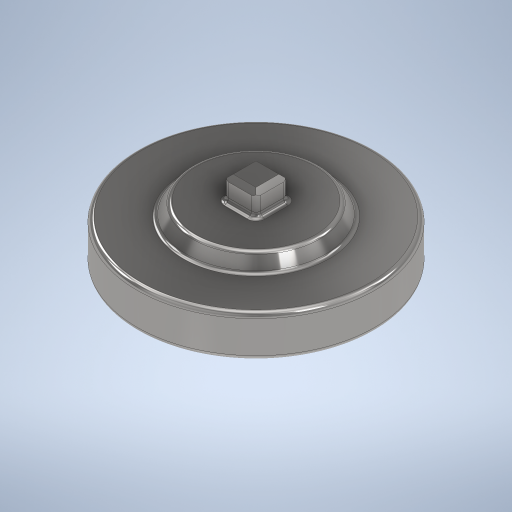
# Autodesk Inventor part: Disc
Saved by Autodesk Inventor 2024 (Build 280153000, 153)
## iProperties
Created: 2024-03-23
Part Number: Disc
Material: Generic
Document SubType Name: Sheet Metal
Designer: MSI-C
Density: 1 g/cm^3
Sheet Metal Rule: Default_mm
Appearance: Steel - Polished
Mass: 22.3559 g
Surface Area: 62.1848 cm^2
Volume: 22.3559 cm^3
Author: MSI-C
Autodesk Inventor part; units mm, degrees
ref_plane "YZ Plane" through (0, 0, 0) normal (1, 0, 0) x (0, 1, 0)
ref_plane "XZ Plane" through (0, 0, 0) normal (0, 1, 0) x (-1, 0, 0)
ref_plane "XY Plane" through (0, 0, 0) normal (0, 0, 1) x (1, 0, 0)
sketch "Sketch1" plane through (0, 0, 0) normal (0, 0, 1) x (1, 0, 0)
  line L0 (0, 0) -> (-5, 0)
  line L1 (-5, 0) -> (-5, 14)
  line L2 (-5, 14) -> (-26, 14)
  line L3 (-26, 14) -> (-26, 23)
  line L4 (-26, 23) -> (-15.5, 23)
  line L5 (-15.5, 23) -> (-13.5, 26)
  line L6 (-13.5, 26) -> (0, 26)
  line L7 (0, 26) -> (0, 0) construction
  line L8 (0, 26) -> (0, 0)
  dimension "d0" = 5
  dimension "d1" = 14
  dimension "d2" = 9
  dimension "d4" = 3
  dimension "d5" = 13.5
  dimension "d6" = 15.5
  dimension "d7" = 26
  dimension "d8" = 26
  constraints: 18 end point, 5 perpendicular, 2 horizontal, 2 vertical, 1 point on line
  measures "d0" distance of L0.start L0.end
  measures "d1" distance of L0.end L1.end
  measures "d2" distance of L2.end L3.end
  measures "d4" vertical distance of L4.end L5.end
  measures "d5" distance of L5.end L6.end
  measures "d6" horizontal distance of L6.end L4.end
  measures "d7" distance from line of L7 L2.end
  measures "d8" distance of L7.start L0.start
revolve "Revolution1" add sketch "Sketch1" angle 360 about axis through (0, 26, 0) along (0, -1, 0)
sketch "Sketch4" plane through (0, 26, 0) normal (0, 1, 0) x (1, 0, 0)
  line L0 (3.5, 3.5) -> (-3.5, 3.5)
  line L1 (-3.5, 3.5) -> (-3.5, -3.5)
  line L2 (-3.5, -3.5) -> (3.5, -3.5)
  line L3 (3.5, -3.5) -> (3.5, 3.5)
  line L4 (3.5, 3.5) -> (-3.5, -3.5) construction
  line L5 (-3.5, 3.5) -> (3.5, -3.5) construction
  point P0 (0, 0)
  dimension "d26" = 7
  dimension "d27" = 7
  constraints: 12 end point, 2 midpoint, 2 parallel, 1 horizontal, 1 perpendicular
  measures "d26" distance of L0.start L0.end
  measures "d27" distance of L2.end L0.start
extrude "Extrusion1" add sketch "Sketch4" along normal blind 5
thread "Thread1" size "M10x1.5" class "6g" standard "ISO Metric profile" length 9
chamfer "Chamfer1" distance 1 angle 45 5 edges at (5, 0, 0) (3.5, 31, 0) (0, 31, 3.5) (-3.5, 31, 0) (0, 31, -3.5)
fillet "Fillet4" radius 1 13 edges at (13.5, 26, 0) (15.5, 23, 0) (26, 23, 0) (26, 14, 0) (5, 14, 0) (3.5, 28, -3.5) (3.5, 28, 3.5) (-3.5, 28, -3.5) (-3.5, 28, 3.5) (3.5, 26, 0) (0, 26, 3.5) (-3.5, 26, 0) (0, 26, -3.5)
sketch "Sketch5" plane through (0, 23, 0) normal (0, 1, 0) x (1, 0, 0)
  point P0 (0, 0)
equation "\"BendRadius\" = Thickness"
equation "\"BendReliefWidth\" = Thickness"
equation "\"BendReliefDepth\" = 0.5 * Thickness"
equation "\"CornerReliefSize\" = 4 * Thickness"
equation "\"MinimumRemnant\" = 2 * Thickness"
equation "\"TransitionRadius\" = BendRadius"
equation "\"JacobiRadiusSize\" = BendRadius"
equation "\"GapSize\" = Thickness"
equation "\"Thickness\" = 0.5"
body "Solid1"
